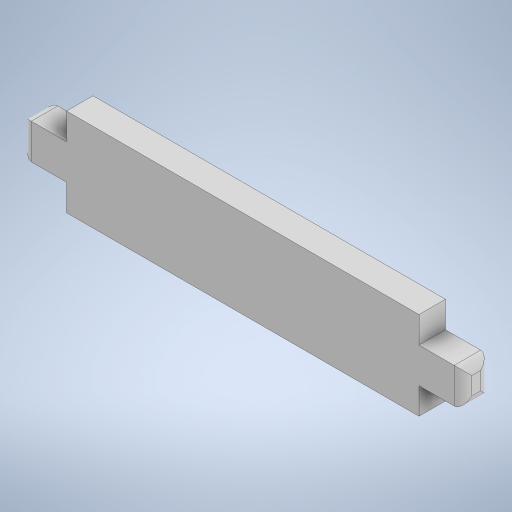
# Autodesk Inventor part: 刃
Saved by Autodesk Inventor 2024.3 (Build 283343000, 343)
## iProperties
Created: 2024-10-08
Part Number: 刃
Material: 一般
Document SubType Name: Modeling
Designer: hikou
Density: 1 g/cm^3
Appearance: 既定
Author: hikou
Autodesk Inventor part; units mm, degrees
ref_plane "YZ Plane" through (0, 0, 0) normal (1, 0, 0) x (0, 1, 0)
ref_plane "XZ Plane" through (0, 0, 0) normal (0, 1, 0) x (-1, 0, 0)
ref_plane "XY Plane" through (0, 0, 0) normal (0, 0, 1) x (1, 0, 0)
sketch "スケッチ1" plane through (0, 0, 0) normal (0, 0, 1) x (1, 0, 0)
  line L0 (-20, -5) -> (20, -5)
  line L1 (20, -5) -> (20, 5)
  line L2 (20, 5) -> (-20, 5)
  line L3 (-20, 5) -> (-20, -5)
  line L4 (-20, -5) -> (20, 5) construction
  line L5 (20, -5) -> (-20, 5) construction
  point P0 (0, 0)
  dimension "d0" = 40
  dimension "d1" = 10
  constraints: 12 end point, 2 midpoint, 2 parallel, 1 horizontal, 1 perpendicular
  measures "d0" distance of L1.end L2.end
  measures "d1" distance of L0.end L1.end
extrude "押し出し1" add sketch "スケッチ1" along normal mid plane 3
sketch "スケッチ2" plane through (-20, -5, 1.5) normal (-1, 0, 0) x (0, 0, 1)
  line L0 (0, 0) -> (0, 10) projected
  line L1 (-3, 3) -> (0, 3)
  line L2 (0, 3) -> (0, 7)
  line L3 (0, 7) -> (-3, 7)
  line L4 (-3, 7) -> (-3, 3)
  line L5 (-3, 3) -> (0, 7) construction
  line L6 (0, 3) -> (-3, 7) construction
  point P0 (-1.5, 5)
  dimension "d4" = 4
  constraints: 12 end point, 2 midpoint, 2 parallel, 1 horizontal, 1 perpendicular, 1 point on line
  measures "d4" distance between parallel lines of L1 L3
extrude "押し出し2" add sketch "スケッチ2" along normal blind 5
sketch "スケッチ3" plane through (20, -5, 1.5) normal (1, 0, 0) x (0, 0, -1)
  line L0 (3, 7) -> (0, 7) projected
  line L1 (0, 3) -> (3, 3) projected
  line L2 (3, 10) -> (0, 10) projected
  line L3 (0, 0) -> (0, 10) projected
  line L4 (0, 0) -> (3, 0) projected
  line L5 (3, 10) -> (3, 0) projected
  point P0 (1.5, 5)
extrude "押し出し3" add sketch "スケッチ3" along normal blind 5 contours L5 L1 L3 L0
fillet "フィレット1" radius 1 8 edges at (25, 2, 0) (25, 0, 1.5) (25, 0, -1.5) (25, -2, 0) (-25, 0, 1.5) (-25, 0, -1.5) (-25, 2, 0) (-25, -2, 0)
